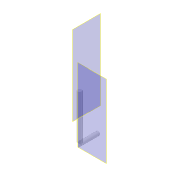
# Autodesk Inventor part: 00_opticalpath
Saved by Autodesk Inventor 2019.4 (Build 234330000, 330)
## iProperties
Created: 2020-11-20
Part Number: 00_opticalpath
Material: Generic
Document SubType Name: Modeling
Designer: diederichbenedict
Density: 1 g/cm^3
Appearance: Polycarbonate - Clear
Author: diederichbenedict
Autodesk Inventor part; units mm, degrees
ref_plane "YZ Plane" through (0, 0, 0) normal (1, 0, 0) x (0, 1, 0)
ref_plane "XZ Plane" through (0, 0, 0) normal (0, 1, 0) x (-1, 0, 0)
ref_plane "XY Plane" through (0, 0, 0) normal (0, 0, 1) x (1, 0, 0)
ref_plane "Work Plane1" through (15.2715, 198.3363, -46.0983) normal (-1, 0, 0) x (0, 1, 0)
sketch "Sketch1" plane through (15.2715, 198.3363, -46.0983) normal (-1, 0, 0) x (0, 1, 0)
  line L0 (-57.2075, -5.2313) -> (-57.2075, -7.2313)
  line L1 (-59.3325, 28.2487) -> (-59.3325, 9.0387)
  line L2 (-39.0825, 28.2487) -> (-39.0825, 9.0387)
  line L3 (-60.777, -7.2313) -> (-38.43, -7.2313) projected
  line L4 (-38.43, -0.2313) -> (-60.777, -0.2313) projected
  line L5 (-113.6123, 22.7696) -> (-98.1523, 22.7696) projected
  line L6 (-105.2077, 22.7696) -> (-105.2077, -2.2304)
  line L7 (-105.2077, -2.2304) -> (-42.2077, -2.2304)
  point P0 (-198.3363, -46.0983)
  dimension "d0" = 25
  dimension "d1" = 63
  constraints: 10 end point, 4 vertical, 1 perpendicular, 1 point on line, 6 other
  measures "d0" distance between parallel lines of L7 L5
  measures "d1" distance from line of L7.end L6
ref_plane "Work Plane2" through (20.8129, 75.0546, -60.4371) normal (0, 0, -1) x (-1, 0, 0)
sketch "Sketch2" plane through (20.8129, 75.0546, -60.4371) normal (0, 0, -1) x (-1, 0, 0)
  circle A0 centre (0.9353, 17.3993) radius 7.73 projected
  circle A1 centre (0.9353, 17.3993) radius 2.641
  point P0 (20.8129, -75.0546)
  constraints: 1 centre point, 1 coincident
sweep "Sweep1" add profiles "Sketch2" path "Sketch1" path curves L6 L7 contours A1
sketch "Sketch3" plane through (15.2715, 198.3363, -46.0983) normal (-1, 0, 0) x (0, 1, 0)
  line L0 (-42.2077, -5.5462) -> (-42.2077, -0.2641) projected
  line L1 (-105.8823, -2.9051) -> (-105.8823, -2.9051) projected
  line L2 (-105.8823, -2.9051) -> (-105.8823, -2.9051) projected
  line L3 (-108.5234, 22.7696) -> (-103.2413, 22.7696) projected
  line L4 (-113.9183, 5.1309) -> (-96.4131, -12.3743)
  line L5 (-96.4131, -12.3743) -> (-115.0261, -30.9873)
  line L6 (-115.0261, -30.9873) -> (-132.5313, -13.4821)
  line L7 (-132.5313, -13.4821) -> (-113.9183, 5.1309)
  line L8 (-113.9183, 5.1309) -> (-89.1622, 5.1309) construction
  line L9 (-105.8823, 22.7696) -> (-105.8823, -27.9051)
  line L10 (-105.8823, -2.9051) -> (-105.8823, -2.9051) projected
  line L11 (-105.8823, -2.9051) -> (-105.8823, -2.9051) projected
  point P0 (-198.3363, -46.0983)
  dimension "d4" = 45
  constraints: 12 end point, 2 parallel, 1 equal length, 1 horizontal, 1 midpoint, 1 perpendicular, 1 point on line, 1 vertical
  measures "d4" angle of L4 L8
extrude "Extrusion1" cut sketch "Sketch3" along normal mid plane 10
sketch "Sketch4" plane through (19.8776, 92.454, -43.1932) normal (0, -0.7071, 0.7071) x (1, 0, 0)
  ellipse E0 centre (0, 0) end of major axis (0, -3.735) minor radius 2.641 (0.3939, 3.6932) -> (-2.641, 0) ccw projected
  ellipse E1 centre (0, 0) end of major axis (0, 3.735) minor radius 2.641 (-2.641, 0) -> (0.3939, -3.6932) ccw projected
  circle A0 centre (0, 0) radius 1.9322
  point P0 (-19.8776, -34.8326)
  point P1 (2.641, 0)
  constraints: 1 centre point, 1 coincident, 2 other
extrude "Extrusion2" cut sketch "Sketch4" against normal blind 10
body "Solid1"
